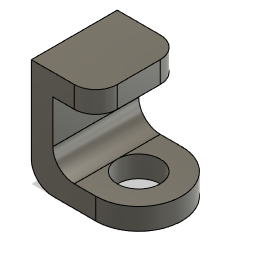
ex3 (Autodesk Fusion 360 design; units mm, degrees)
Autodesk Fusion 360 part; units mm, degrees
note: some values were not read from the file. Set by a fixed rule: which sketch regions a step uses.
sketch "Sketch1" plane through (0, 0, 0) normal (0, 1, 0) x (1, 0, 0)
  line L0 (0, 0) -> (0, 40)
  line L1 (0, 20) -> (30, 20)
  circle A0 centre (30, 20) radius 10
  circle A1 centre (30, 20) radius 20
  line L2 (0, 40) -> (30, 40)
  line L3 (0, 0) -> (30, 0)
  line L4 (0, 40) -> (10, 40)
  line L5 (10, 0) -> (10, 40)
  line L6 (10, 0) -> (0, 0)
  line L7 (30, 40) -> (30, 0)
  dimension "d1" = 40
  dimension "d3" = 20
  dimension "d4" = 10
  constraint coincident L0.start L3.start
  constraint vertical L0
  constraint midpoint L0 L1.start
  constraint perpendicular L0 L1
  constraint coincident L1.end A0.centre
  constraint concentric A0 A1
  constraint coincident A1 L2.end
  constraint tangent A1 L2
  constraint perpendicular L0 L2
  constraint coincident A1 L3.end
  constraint tangent A1 L3
  constraint coincident L2 L4.end
  constraint coincident L3 L5.start
  constraint perpendicular L4 L5
  measures "d1" distance of L0.start L0.end
  measures "d3" diameter of A0
  measures "d4" distance of L0.end L4.end
extrude "Extrude1" add sketch "Sketch1" along normal blind 50.06 contours L0 L1 L3 L5 L6 | L0 L1 L2 L4 L5
extrude "Extrude2" add sketch "Sketch1" along normal blind 10 contours A1 L3 L5 | L1 A0 A1 L7 | A1 L2 L5 | L1 A0 A1 L7 | A0 A1 L7
sketch "Sketch2" plane through (0, 50.06, 0) normal (0, 1, 0) x (-1, 0, 0)
  line L0 (-10, 0) -> (-10, -40)
  line L1 (-10, -40) -> (0, -40)
  line L2 (0, -40) -> (0, 0)
  line L3 (0, 0) -> (-10, 0)
  line L4 (0, -40) -> (-30, -40)
  line L5 (-30, -40) -> (-30, 0)
  line L6 (-30, 0) -> (0, 0)
  constraint coincident L1.end L2.start
  constraint perpendicular L2 L4
  constraint perpendicular L4 L5
  constraint coincident L2.end L3.start
  constraint perpendicular L2 L6
extrude "Extrude3" add sketch "Sketch2" against normal blind 10 contours L0 L4 L5 L6
fillet "Fillet1" radius 10 4 edges at (10, 10, -20) (0, 0, -20) (30, 45.06, 0) (30, 45.06, -40)
